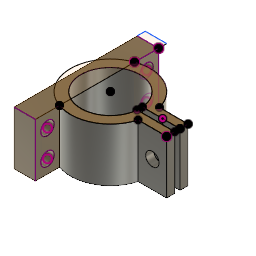
bearing_holder (Autodesk Fusion 360 design; units mm, degrees)
Autodesk Fusion 360 part; units mm, degrees
note: some values were not read from the file. Chosen so that the rebuilt part matches the saved one: that a step has no effect. Set by a fixed rule: which sketch regions a step uses.
sketch "Sketch1" plane through (0, 0, 0) normal (0, 0, 1) x (1, 0, 0)
  line L0 (0, 40) -> (0, 0)
  line L1 (23.9533, 21.0123) -> (31.5, 21.0123)
  line L2 (31.5, 24.0123) -> (27.3144, 24.0123)
  line L3 (23.9545, 19) -> (31.5, 19)
  line L4 (31.5, 16) -> (27.3178, 16)
  line L5 (8, 0) -> (8, 6)
  line L6 (8, 34) -> (8, 40)
  arc A0 (23.9533, 21.0123) -> (23.9545, 19) centre (13, 20) ccw
  arc A1 (8, 6) -> (27.3178, 16) centre (13, 20) ccw
  arc A2 (27.3144, 24.0123) -> (8, 34) centre (13, 20) ccw
  line L7 (8, 6) -> (8, 0)
  line L8 (8, 6) -> (8, 0)
  line L9 (0, 0) -> (0, -3)
  line L10 (0, -3) -> (8, -3)
  line L11 (8, -3) -> (8, 0)
  line L12 (0, 40) -> (0, 43)
  line L13 (0, 43) -> (8, 43)
  line L14 (8, 43) -> (8, 40)
  line L15 (31.5, 24.0123) -> (38, 24.0123)
  line L16 (38, 24.0123) -> (38, 21)
  line L17 (38, 21) -> (31.5, 21)
  line L18 (31.5, 21) -> (31.5, 21.0123)
  line L19 (31.5, 16) -> (38, 16)
  line L20 (38, 16) -> (38, 19)
  line L21 (38, 19) -> (31.5, 19)
  point P0 (26, 20)
  point P1 (26, 20)
  point P2 (22.5, 21)
  dimension "d1" = 8
  dimension "d4" = 3
  dimension "d5" = 3
  dimension "d30" = 22
  dimension "d31" = 3
  constraint vertical L5
  constraint vertical L0
  constraint coincident L0.end L9.start
  constraint coincident P1 P0
  constraint horizontal L1
  constraint horizontal L2
  constraint horizontal L3
  constraint horizontal L4
  constraint coincident L6.start A1
  constraint coincident L2.end A1
  constraint vertical L9
  constraint horizontal L10
  constraint vertical L11
  constraint vertical L12
  constraint horizontal L13
  constraint vertical L14
  constraint horizontal L15
  constraint vertical L16
  constraint horizontal L17
  constraint vertical L18
  constraint horizontal L19
  constraint vertical L20
  constraint horizontal L21
  measures "d1" distance of L0.end L5.start
  measures "d4" distance of L1.end L2.start
  measures "d5" distance of L3.end L4.start
  measures "d30" diameter of A0
  measures "d31" distance of L6.end L13.end
extrude "Extrude1" add sketch "Sketch1" along normal blind 20
sketch "Sketch2" plane through (8, 0, 0) normal (1, 0, 0) x (0, 1, 0)
  line L0 (0, 0) -> (8, 0)
  line L1 (8, 0) -> (8, 20)
  line L2 (8, 20) -> (0, 20)
  line L3 (0, 20) -> (0, 0)
  line L4 (4, 20) -> (4, 10)
  line L5 (4, 10) -> (4, 15)
  circle A0 centre (4, 15) radius 2.5
  line L6 (4, 0) -> (4, 10)
  circle A1 centre (4, 5) radius 2.5
  line L7 (32, 0) -> (40, 0)
  line L8 (36, 0) -> (36, 10)
  circle A2 centre (36, 5) radius 2.5
  line L9 (32, 20) -> (40, 20)
  line L10 (36, 20) -> (36, 10)
  circle A3 centre (36, 15) radius 2.5
  dimension "d8" = 5
  dimension "d9" = 5
  dimension "d10" = 10
  dimension "d11" = 5
  dimension "d12" = 10
  dimension "d13" = 5
  constraint midpoint L2 L4.start
  constraint perpendicular L2 L4
  constraint midpoint L4 L5.end
  constraint coincident L5.end A0.centre
  constraint midpoint L0 L6.start
  constraint midpoint L6 A1.centre
  constraint midpoint L7 L8.start
  constraint perpendicular L7 L8
  constraint midpoint L8 A2.centre
  constraint midpoint L9 L10.start
  constraint perpendicular L9 L10
  constraint midpoint L10 A3.centre
  measures "d8" diameter of A0
  measures "d9" diameter of A1
  measures "d10" distance of L8.start L8.end
  measures "d11" diameter of A2
  measures "d12" distance of L10.start L8.end
  measures "d13" diameter of A3
sketch "Sketch13" plane through (0, 0, 0) normal (-1, 0, 0) x (0, -1, 0)
  line L0 (-43, 0) -> (3, 0)
  line L1 (3, 0) -> (3, 20)
  line L2 (3, 20) -> (-43, 20)
  line L3 (-43, 20) -> (-43, 0)
  line L4 (-34, 20) -> (-43, 20)
  line L5 (-34, 0) -> (-43, 0)
  line L6 (-38.5, 20) -> (-38.5, 0)
  circle A0 centre (-38.5, 15.0002) radius 2.5
  circle A1 centre (-38.5, 4.9568) radius 2.5
  line L7 (3, 20) -> (-6, 20)
  line L8 (3, 0) -> (-6, 0)
  line L9 (-1.5, 20) -> (-1.5, 0)
  circle A2 centre (-1.5, 14.9561) radius 2.5
  circle A3 centre (-1.5, 5.0194) radius 2.5
  dimension "d32" = 5
  dimension "d33" = 5
  dimension "d34" = 5
  dimension "d35" = 5
  constraint midpoint L4 L6.start
  constraint midpoint L5 L6.end
  constraint coincident L6 A0.centre
  constraint coincident L6 A1.centre
  constraint midpoint L7 L9.start
  constraint midpoint L8 L9.end
  constraint coincident L9 A2.centre
  constraint coincident L9 A3.centre
  measures "d32" diameter of A0
  measures "d33" diameter of A1
  measures "d34" diameter of A2
  measures "d35" diameter of A3
sketch "Sketch12" plane through (0, 0, 20) normal (0, 0, 1) x (-1, 0, 0)
  line L0 (-23.9533, -21.0123) -> (-31.5, -21.0123)
  line L1 (-38, -24.0123) -> (-27.3144, -24.0123)
  arc A0 (-27.3144, -24.0123) -> (-8, -34) centre (-13, -20) ccw
  line L2 (-8, -34) -> (-8, -43)
  line L3 (0, -43) -> (0, 3)
  line L4 (-8, 3) -> (-8, -6)
  arc A1 (-8, -6) -> (-27.3178, -16) centre (-13, -20) ccw
  line L5 (-27.3178, -16) -> (-38, -16)
  line L6 (-38, -19) -> (-23.9545, -19)
  arc A2 (-23.9533, -21.0123) -> (-23.9545, -19) centre (-13, -20) ccw
  line L7 (-8, -43) -> (0, -43)
  line L8 (0, -43) -> (0, -46)
  line L9 (0, -46) -> (-8, -46)
  line L10 (-8, -46) -> (-8, -43)
  line L11 (0, 3) -> (-8, 3)
  line L12 (-8, -43) -> (0, -43)
  line L13 (-38, -16) -> (-38, -19)
  line L14 (-31.5, -21.0123) -> (-31.5, -21)
  line L15 (-31.5, -21) -> (-38, -21)
  line L16 (-38, -21) -> (-38, -24.0123)
  constraint horizontal L7
  constraint vertical L8
  constraint horizontal L9
  constraint vertical L10
  constraint coincident L2.end L7.start
extrude "Extrude2" [no effect]
extrude "Extrude9" cut sketch "Sketch13" against normal blind 10 contours L6 A1 | L6 A1 | L6 A0 | L6 A0 | L9 A3 | L9 A3 | L9 A2 | L9 A2
sketch "Sketch11" plane through (8, 0, 0) normal (1, 0, 0) x (0, 1, 0)
  line L0 (34, 20) -> (34, 0)
  line L1 (34, 0) -> (43, 0)
  line L2 (43, 20) -> (34, 20)
  circle A0 centre (38.5, 15.0002) radius 2.5
  circle A1 centre (38.5, 4.9568) radius 2.5
  line L3 (43, 0) -> (43, 20)
sketch "Sketch10" plane through (8, 0, 0) normal (1, 0, 0) x (0, 1, 0)
  line L0 (6, 20) -> (-3, 20)
  line L1 (-3, 0) -> (6, 0)
  line L2 (6, 0) -> (6, 20)
  circle A0 centre (1.5, 5.0194) radius 2.5
  circle A1 centre (1.5, 14.9561) radius 2.5
  line L3 (-3, 20) -> (-3, 0)
sketch "Sketch9" plane through (0, 0, 20) normal (0, 0, 1) x (-1, 0, 0)
  line L0 (0, -43) -> (0, 3)
  line L1 (-8, 3) -> (-8, -6)
  line L2 (-27.3178, -16) -> (-38, -16)
  line L3 (-38, -19) -> (-23.9545, -19)
  line L4 (-23.9533, -21.0123) -> (-31.5, -21.0123)
  line L5 (-38, -24.0123) -> (-27.3144, -24.0123)
  arc A0 (-8, -6) -> (-27.3178, -16) centre (-13, -20) ccw
  arc A1 (-23.9533, -21.0123) -> (-23.9545, -19) centre (-13, -20) ccw
  arc A2 (-27.3144, -24.0123) -> (-8, -34) centre (-13, -20) ccw
  line L6 (-8, -34) -> (-8, -43)
  line L7 (0, 3) -> (-8, 3)
  line L8 (-8, -43) -> (0, -43)
  line L9 (-38, -16) -> (-38, -19)
  line L10 (-31.5, -21.0123) -> (-31.5, -21)
  line L11 (-31.5, -21) -> (-38, -21)
  line L12 (-38, -21) -> (-38, -24.0123)
sketch "Sketch15" plane through (0, 16, 0) normal (0, -1, 0) x (1, 0, 0)
  line L0 (27.3178, 0) -> (38, 0)
  line L1 (38, 0) -> (38, 20)
  line L2 (38, 20) -> (27.3178, 20)
  line L3 (27.3178, 20) -> (27.3178, 0)
  circle A0 centre (32.6589, 10) radius 2.5
  dimension "d39" = 5
  measures "d39" diameter of A0
extrude "Extrude10" cut sketch "Sketch15" against normal blind 6 contours A0
extrude "Extrude11" cut 1 faces at (32.1232, 22, 11.0657) along direction (0, 1, 0) blind 10
sketch "Sketch16" plane through (8, 0, 0) normal (1, 0, 0) x (0, 1, 0)
sketch "Sketch17" plane through (0, -3, 0) normal (0, -1, 0) x (1, 0, 0)
  line L0 (0, 0) -> (8, 0)
  line L1 (8, 0) -> (8, 20)
  line L2 (8, 20) -> (0, 20)
  line L3 (0, 20) -> (0, 0)
sketch "Sketch18" plane through (4, -3, 10) normal (0, -1, 0) x (1, 0, 0)
sketch "Sketch19" plane through (0, 0, 20) normal (0, 0, 1) x (-1, 0, 0)
  line L0 (-8, -34) -> (-8, -43)
  line L1 (-8, -6) -> (-8, -34)
  point P0 (-8, -6)
  point P1 (-8, -34)
  constraint coincident P0 L1.start
  constraint coincident P1 L0.start
sketch "Sketch20" plane through (0, 0, 20) normal (0, 0, 1) x (1, 0, 0)
  line L0 (8, 34) -> (8, 43)
  line L1 (8, 6) -> (8, 34)
  line L2 (8, 6) -> (8, 34)
  line L3 (38, 16) -> (38, 19)
  line L4 (27.3178, 16) -> (38, 16)
  line L5 (38, 19) -> (38, 16)
  line L6 (38, 19) -> (23.9545, 19)
  line L7 (23.9533, 21.0123) -> (38, 21)
  line L8 (38, 21) -> (38, 24.0123)
  line L9 (38, 24.0123) -> (38, 21)
  line L10 (38, 24.0123) -> (27.3144, 24.0123)
  arc A0 (27.3144, 24.0123) -> (27.3178, 16) centre (13, 20) ccw
  arc A1 (23.9533, 21.0123) -> (23.9545, 19) centre (13, 20) ccw
  point P0 (8, 6)
  point P1 (8, 34)
  point P2 (13, 20)
  point P3 (38, 16)
  point P4 (38, 16)
  point P5 (38, 21)
  point P6 (38, 24.0123)
  point P7 (38, 24.0123)
  constraint coincident P0 L1.start
  constraint coincident P1 L0.start
  constraint coincident P2 A0.centre
  constraint coincident L4.start A0.end
  constraint coincident P4 P3
  constraint coincident L3.end L5.start
  constraint coincident L6.end A1.end
  constraint coincident L7.start A1.start
  constraint coincident P5 L7.end
  constraint coincident P7 P6
  constraint coincident L10.end A0.start
sketch "Sketch14" plane through (0, 16, 0) normal (0, -1, 0) x (1, 0, 0)
  line L0 (27.3178, 0) -> (38, 0)
  line L1 (38, 20) -> (27.3178, 20)
  line L2 (27.3178, 20) -> (27.3178, 0)
  circle A0 centre (29.4089, 10) radius 2.5
  line L3 (38, 0) -> (38, 20)
  dimension "d38" = 5
  measures "d38" diameter of A0
sketch "Sketch3" plane through (0, 0, 20) normal (0, 0, 1) x (-1, 0, 0)
  line L0 (-23.9533, -21.0123) -> (-31.5, -21.0123)
  line L1 (-38, -24.0123) -> (-27.3144, -24.0123)
  line L2 (-27.3178, -16) -> (-38, -16)
  line L3 (-38, -19) -> (-23.9545, -19)
  line L4 (-4, 0) -> (-4, -40)
  arc A0 (-8, -6) -> (-27.3178, -16) centre (-13, -20) ccw
  line L5 (0, -43) -> (0, 3)
  line L6 (-8, 3) -> (-8, -6)
  arc A1 (-23.9533, -21.0123) -> (-23.9545, -19) centre (-13, -20) ccw
  arc A2 (-27.3144, -24.0123) -> (-8, -34) centre (-13, -20) ccw
  line L7 (-8, -34) -> (-8, -43)
  line L8 (0, 3) -> (-8, 3)
  line L9 (-8, -43) -> (0, -43)
  line L10 (-38, -16) -> (-38, -19)
  line L11 (-31.5, -21.0123) -> (-31.5, -21)
  line L12 (-31.5, -21) -> (-38, -21)
  line L13 (-38, -21) -> (-38, -24.0123)
extrude "Extrude3" [suppressed]
sketch "Sketch4" plane through (0, 16, 0) normal (0, -1, 0) x (1, 0, 0)
  line L0 (27.3178, 0) -> (31.5, 0)
  line L1 (31.5, 0) -> (31.5, 20)
  line L2 (31.5, 20) -> (27.3178, 20)
  line L3 (29.4089, 20) -> (29.4089, 0)
  circle A0 centre (29.4089, 10) radius 2.5
  line L4 (27.3178, 20) -> (27.3178, 0)
  dimension "d18" = 5
  constraint midpoint L2 L3.start
  constraint midpoint L0 L3.end
  constraint midpoint L3 A0.centre
  measures "d18" diameter of A0
extrude "Extrude4" [suppressed]
sketch "Sketch5" plane through (0, 0, 20) normal (0, 0, 1) x (-1, 0, 0)
  line L0 (-27.3178, -16) -> (-31.5, -16)
  line L1 (-31.5, -16) -> (-31.5, -19)
  line L2 (-31.5, -19) -> (-23.9545, -19)
  line L3 (-23.9533, -21.0123) -> (-31.5, -21.0123)
  line L4 (-31.5, -21.0123) -> (-31.5, -24.0123)
  line L5 (-31.5, -24.0123) -> (-27.3144, -24.0123)
  line L6 (-15.3559, -18.2409) -> (-23.9533, -21.0123)
  line L7 (-27.3178, -16) -> (-15.2294, -16)
  arc A0 (-15.3559, -18.2409) -> (-15.2294, -16) centre (-13.0622, -17.2464) ccw
  arc A1 (-8, -6) -> (-27.3178, -16) centre (-13, -20) ccw
  line L8 (-8, 3) -> (-8, -6)
  arc A2 (-23.9533, -21.0123) -> (-23.9545, -19) centre (-13, -20) ccw
  arc A3 (-27.3144, -24.0123) -> (-8, -34) centre (-13, -20) ccw
  line L9 (-8, -34) -> (-8, -43)
  line L10 (0, -43) -> (0, 3)
  line L11 (0, 3) -> (-8, 3)
  line L12 (-8, -43) -> (0, -43)
  dimension "d21" = 5
  constraint coincident L3.start L6.end
  constraint coincident L0.start L7.start
  constraint parallel L2 L7
  measures "d21" diameter of A0
extrude "Extrude5" [suppressed]
sketch "Sketch6" plane through (-3.8811, 12.0396, 0) normal (0.306812, -0.95177, 0) x (0.95177, 0.306812, 0)
  line L0 (29.2449, 20) -> (20.2118, 20)
  line L1 (20.2118, 20) -> (20.2118, 0)
  line L2 (20.2118, 0) -> (29.2449, 0)
  line L3 (29.2449, 0) -> (29.2449, 20)
sketch "Sketch7" plane through (0, 40, 0) normal (0, 1, 0) x (-1, 0, 0)
  line L0 (-4, 0) -> (-4, 20)
  line L1 (-4, 20) -> (-8, 20)
  line L2 (-8, 0) -> (-4, 0)
  line L3 (-4, 20) -> (-8, 20)
  line L4 (-8, 20) -> (-8, 0)
  line L5 (-8, 0) -> (-4, 0)
  line L6 (-4, 0) -> (-4, 20)
  line L7 (-4, 20) -> (-8, 20)
  line L8 (-8, 20) -> (-8, 0)
  line L9 (-8, 0) -> (-4, 0)
  line L10 (-4, 0) -> (-4, 20)
  line L11 (-8, 20) -> (-8, 0)
  constraint horizontal L3
  constraint vertical L4
  constraint horizontal L5
  constraint vertical L6
  constraint coincident L2.start L4.end
  constraint coincident L0.end L1.start
  constraint horizontal L7
  constraint vertical L8
  constraint horizontal L9
  constraint vertical L10
extrude "Extrude7" [suppressed]
extrude "Extrude6" [suppressed]
sketch "Sketch8" plane through (0, 0, 20) normal (0, 0, 1) x (-1, 0, 0)
  line L0 (-27.3178, -16) -> (-31.5, -16)
  line L1 (-31.5, -16) -> (-31.5, -19)
  line L2 (-31.5, -19) -> (-23.9545, -19)
  arc A0 (-8, -6) -> (-27.3178, -16) centre (-13, -20) ccw
  line L3 (-8, 3) -> (-8, -6)
  arc A1 (-23.9533, -21.0123) -> (-23.9545, -19) centre (-13, -20) ccw
  line L4 (0, -43) -> (0, 3)
  line L5 (0, 3) -> (-8, 3)
  line L6 (-23.9533, -21.0123) -> (-31.5, -21.0123)
  line L7 (-31.5, -21.0123) -> (-31.5, -24.0123)
  line L8 (-31.5, -24.0123) -> (-27.3144, -24.0123)
  arc A2 (-27.3144, -24.0123) -> (-8, -34) centre (-13, -20) ccw
  line L9 (-8, -34) -> (-8, -43)
  line L10 (-8, -43) -> (0, -43)
extrude "Extrude8" [suppressed]
